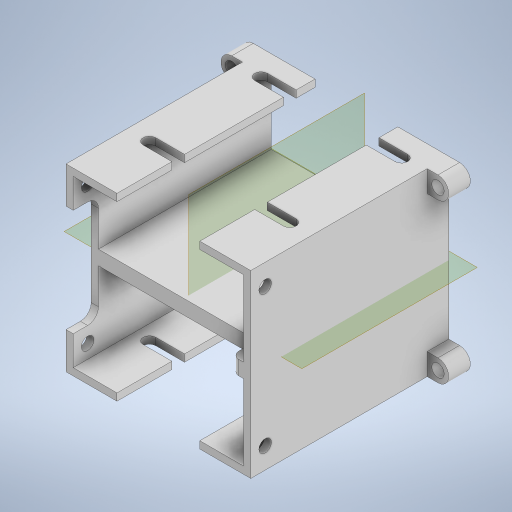
# Autodesk Inventor part: POUPLY_P1_moteur
Saved by Autodesk Inventor 2024 (Build 280153000, 153)
## iProperties
Created: 2024-02-11
Part Number: POUPLY_P1_moteur
Material: Generic
Document SubType Name: Sheet Metal
Designer: luc4s
Density: 1 g/cm^3
Appearance: Default
Sheet Metal Rule: Default
Author: luc4s
## iProperties of the stored document POUPLY_P1_moteur_3DPrint.ipt
Created: 2024-02-11
Part Number: POUPLY_P1_moteur_3DPrint
Material: Generic
Document SubType Name: Modeling
Designer: luc4s
Density: 1 g/cm^3
Appearance: Default
Author: luc4s
Autodesk Inventor part; units mm, degrees
ref_plane "YZ Plane" through (0, 0, 0) normal (1, 0, 0) x (0, 1, 0)
ref_plane "XZ Plane" through (0, 0, 0) normal (0, 1, 0) x (-1, 0, 0)
ref_plane "XY Plane" through (0, 0, 0) normal (0, 0, 1) x (1, 0, 0)
sketch "Espace_Moteurs" plane through (0, 0, 0) normal (0, 0, 1) x (1, 0, 0)
  line L0 (-11.5, 25) -> (-25.65, 25)
  line L1 (-25.65, 25) -> (-25.65, 0)
  line L2 (-25.65, 0) -> (25.65, 0)
  line L3 (25.65, 0) -> (25.65, 25)
  line L4 (25.65, 25) -> (11.5, 25)
  line L5 (11.5, 25) -> (11.5, 23)
  line L6 (11.5, 23) -> (23.65, 23)
  line L7 (23.65, 23) -> (23.65, 2)
  line L8 (23.65, 2) -> (-23.65, 2)
  line L9 (-23.65, 2) -> (-23.65, 23)
  line L10 (-23.65, 23) -> (-11.5, 23)
  line L11 (-11.5, 23) -> (-11.5, 25)
  line L12 (0, 34.7545) -> (0, 0) construction
  line L13 (0, 0) -> (39.3483, 0) construction
  point P0 (23.65, 12.5)
  point P1 (-18.575, 25)
  point P2 (-17.575, 23)
  dimension "d0" = 25
  dimension "d2" = 2
  dimension "d3" = 2
  dimension "d4" = 2
  dimension "d5" = 2
  dimension "d6" = 2
  dimension "d7" = 12.15
  dimension "d8" = 12.15
  dimension "d9" = 25
  dimension "d76" = 23
  constraints: 28 end point, 10 perpendicular, 3 midpoint, 2 horizontal, 1 parallel, 1 point on line, 1 vertical, 1 other
  measures "d0" distance between parallel lines of L2 L0
  measures "d2" distance from line of L3 point (23.65, 12.5)
  measures "d3" distance between parallel lines of L2 L8
  measures "d4" distance between parallel lines of L1 L9
  measures "d5" vertical distance of point (-18.575, 25) point (-17.575, 23)
  measures "d6" distance between parallel lines of L4 L6
  measures "d7" distance of L9.end L10.end
  measures "d8" distance of L5.end L6.end
  measures "d9" distance of L2.end L3.end
  measures "d76" distance of L5.end L10.end
extrude "Moteur_bloc_1" add sketch "Espace_Moteurs" along normal blind 55
sketch "Bloc_vis_1" plane through (25.65, 0, 0) normal (1, 0, 0) x (0, 0, -1)
  line L0 (0, 25) -> (-55, 25) projected
  line L1 (0, 25) -> (-6, 25)
  line L2 (-6, 25) -> (-6, 19)
  line L3 (-6, 19) -> (0, 19)
  line L4 (0, 19) -> (0, 25)
  point P0 (0, 0)
  dimension "d12" = 6
  dimension "d13" = 6
  constraints: 8 end point, 2 parallel, 1 horizontal, 1 perpendicular
  measures "d12" distance of L1.end L2.end
  measures "d13" distance of L2.end L3.end
extrude "Ext_Bloc_vis_1" add sketch "Bloc_vis_1" along normal blind 6
fillet "Fillet1" radius 3 2 edges at (31.65, 19, 3) (31.65, 25, 3)
ref_plane "Work Plane3" through (0, 0, 0) normal (-1, 0, 0) x (0, 0, 1)
mirror "Mirror3" about plane through (0, 0, 0) normal (-1, 0, 0) of "Ext_Bloc_vis_1"
fillet "Fillet2" radius 3 2 edges at (-31.65, 25, 3) (-31.65, 19, 3)
mirror "Mirror4" about plane through (-25.65, 0, 0) normal (0, -1, 0) of "Moteur_bloc_1", "Ext_Bloc_vis_1", "Mirror3", "Fillet2", "Fillet1"
sketch "Sketch3" plane through (-25.65, 19, 6) normal (0, 0, 1) x (1, 0, 0)
  circle A0 centre (-3, -41) radius 1.75
  line L0 (0, 6) -> (0, -44) projected
  line L1 (0, -44) -> (-3, -44) projected
  point P0 (25.65, -19)
  dimension "d18" = 3
  dimension "d19" = 3
  dimension "d67" = 3.5
  constraints: 1 centre point
  measures "d18" distance from line of A0.centre L0
  measures "d19" distance from line of L1 A0.centre
  measures "d67" diameter of A0
extrude "Extrusion3" cut sketch "Sketch3" against normal blind 6
mirror "Mirror5" about plane through (0, 0, 0) normal (-1, 0, 0) of "Extrusion3"
ref_plane "Work Plane4" through (-28.65, 0, 0) normal (0, -1, 0) x (1, 0, 0)
mirror "Mirror6" about plane through (-28.65, 0, 0) normal (0, -1, 0) of "Extrusion3", "Mirror5"
sketch "Sketch4" plane through (-25.65, 19, 6) normal (-1, 0, 0) x (0, 0, 1)
  circle A0 centre (45, 0.15) radius 1.75
  line L0 (0, 6) -> (49, 6) projected
  line L1 (45, 0.15) -> (45, 4) construction
  line L2 (-6, 4) -> (49, 4) projected
  line L3 (-6, -44) -> (49, -44) projected
  line L4 (0, 6) -> (0, 0) projected
  line L5 (0, -38) -> (0, -44) projected
  point P0 (-6, -19)
  dimension "d22" = 3.5
  dimension "d26" = 45
  constraints: 2 end point, 1 centre point, 1 perpendicular, 1 point on line
  measures "d22" diameter of A0
  measures "d26" distance from line of L4 L1.start
extrude "Extrusion4" cut sketch "Sketch4" against normal blind 55
mirror "Mirror7" about plane through (-28.65, 0, 0) normal (0, -1, 0) of "Extrusion4"
sketch "Sketch6" plane through (-23.65, -2, 0) normal (0, -1, 0) x (1, 0, 0)
  line L0 (47.3, 55) -> (0, 55) projected
  line L1 (0, 55) -> (44, 55)
  line L2 (44, 55) -> (44, 48)
  line L3 (44, 48) -> (0, 48)
  line L4 (0, 48) -> (0, 55)
  point P0 (23.65, 0)
  dimension "d36" = 7
  constraints: 8 end point, 2 parallel, 1 horizontal, 1 perpendicular
  measures "d36" distance between parallel lines of L3 L0
extrude "Extrusion6" cut sketch "Sketch6" against normal blind 4
sketch "Sketch7" plane through (-25.65, 19, 6) normal (-1, 0, 0) x (0, 0, 1)
  line L0 (49, 4) -> (49, -42) projected
  line L1 (49, -4.15) -> (42, -4.15)
  line L2 (42, -4.15) -> (42, -33.85)
  line L3 (42, -33.85) -> (49, -33.85)
  line L4 (49, -33.85) -> (49, -4.15)
  line L5 (0, 6) -> (49, 6) projected
  line L6 (0, -44) -> (49, -44) projected
  point P0 (-6, -19)
  point P1 (49, -33.85)
  dimension "d39" = 10.15
  dimension "d40" = 10.15
  dimension "d41" = 7
  constraints: 8 end point, 2 parallel, 1 horizontal, 1 perpendicular, 1 point on line
  measures "d39" distance from line of L5 L1.start
  measures "d40" distance from line of L6 L3.end
  measures "d41" distance of L1.start L1.end
extrude "Extrusion7" cut sketch "Sketch7" against normal blind 40
fillet "Fillet3" radius 3 1 edges at (-24.65, 14.85, 48)
fillet "Fillet4" radius 3 1 edges at (-24.65, -14.85, 48)
sketch "Sketch9" plane through (-28.65, -25, 0) normal (0, -1, 0) x (1, 0, 0)
  line L0 (17.15, 7) -> (9.15, 7) construction
  line L1 (17.15, 5.25) -> (9.15, 5.25)
  line L2 (9.15, 8.75) -> (17.15, 8.75)
  arc A0 (17.15, 5.25) -> (17.15, 8.75) centre (17.15, 7) ccw
  arc A1 (9.15, 8.75) -> (9.15, 5.25) centre (9.15, 7) ccw
  line L3 (17.15, 0) -> (0, 0) projected
  line L4 (17.15, 0) -> (17.15, 55) projected
  line L5 (13.15, 7) -> (13.15, 38) construction
  line L6 (13.15, 24.25) -> (44.15, 24.25) construction
  line L7 (28.65, 24.25) -> (28.65, -1.049) construction
  point P0 (28.65, 0)
  point P1 (28.65, 49.549)
  dimension "d72" = 1.75
  dimension "d73" = 8
  dimension "d74" = 7
  dimension "d75" = 4
  dimension "d79" = 31
  dimension "d80" = 31
  dimension "d81" = 15.5
  dimension "d82" = 15.5
  constraints: 14 end point, 4 point on circle, 4 tangent, 2 centre point, 2 horizontal, 2 midpoint, 2 vertical, 1 parallel, 1 point on line, 1 symmetric about line
  measures "d72" radius of A0
  measures "d73" distance of L2.start L2.end
  measures "d74" distance from line of L3 L5.start
  measures "d75" distance from line of L4 L5.start
  measures "d79" distance of L5.start L5.end
  measures "d80" distance of L6.start L6.end
  measures "d81" distance between parallel lines of L2 L6
  measures "d82" distance from line of L7 L6.start
extrude "Extrusion10" cut sketch "Sketch9" against normal blind 10
pattern_linear "Rectangular Pattern3" count 2 spacing 31 along (0, 0, 1) count 2 spacing 31 along (1, 0, 0) of "Extrusion10"
sketch "Sketch11" plane through (-25.65, 19, 6) normal (-1, 0, 0) x (0, 0, 1)
  point P0 (-6, -19)
fillet "Fillet5" radius 2 1 edges at (20.35, 0, 48)
fillet "Fillet6" radius 2 1 edges at (20.35, 0, 55)
mirror "Mirror10" about plane through (0, 0, 0) normal (0, 1, 0) of "Extrusion10", "Rectangular Pattern3"
equation "\"BendRadius\" = Thickness"
equation "\"BendReliefWidth\" = Thickness"
equation "\"BendReliefDepth\" = 0.5 * Thickness"
equation "\"CornerReliefSize\" = 4 * Thickness"
equation "\"MinimumRemnant\" = 2 * Thickness"
equation "\"TransitionRadius\" = BendRadius"
equation "\"JacobiRadiusSize\" = BendRadius"
equation "\"GapSize\" = Thickness"
equation "\"Thickness\" = 3.048"
body "Solid1"
